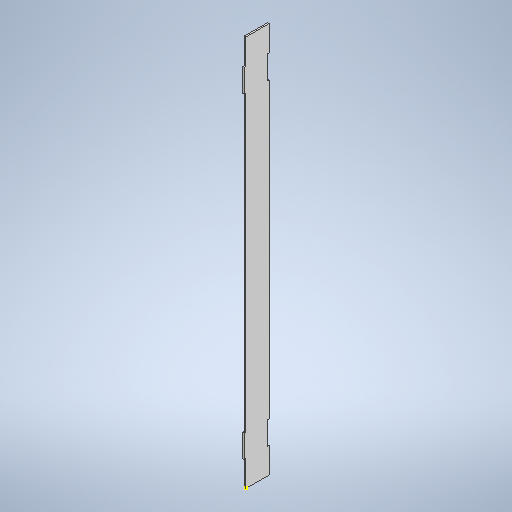
# Autodesk Inventor part: PAREDES LAT-CONTRA
Saved by Autodesk Inventor 2025.2 (Build 292293000, 293)
## iProperties
Created: 2025-05-13
Part Number: PAREDES LAT-CONTRA
Material: Genérico
Document SubType Name: Modeling
Designer: marce
Density: 1 g/cm^3
Appearance: Padrão
Author: marce
Autodesk Inventor part; units mm, degrees
ref_plane "YZ Plane" through (0, 0, 0) normal (1, 0, 0) x (0, 1, 0)
ref_plane "XZ Plane" through (0, 0, 0) normal (0, 1, 0) x (-1, 0, 0)
ref_plane "XY Plane" through (0, 0, 0) normal (0, 0, 1) x (1, 0, 0)
sketch "Esboço1" plane through (0, 0, 0) normal (1, 0, 0) x (0, 1, 0)
  line L0 (1008, 0) -> (1008, -60)
  line L1 (0, -60) -> (0, 0)
  line L2 (1008, 0) -> (942, 0)
  line L3 (942, 0) -> (942, 4)
  line L4 (942, 4) -> (882, 4)
  line L5 (882, 4) -> (882, 0)
  line L6 (0, 0) -> (66, 0)
  line L7 (66, 0) -> (66, 4)
  line L8 (66, 4) -> (126, 4)
  line L9 (126, 4) -> (126, 0)
  line L10 (126, 0) -> (882, 0)
  line L11 (1008, -60) -> (942, -60)
  line L12 (942, -60) -> (942, -56)
  line L13 (942, -56) -> (882, -56)
  line L14 (882, -56) -> (882, -60)
  line L15 (0, -60) -> (66, -60)
  line L16 (66, -60) -> (66, -56)
  line L17 (66, -56) -> (126, -56)
  line L18 (126, -56) -> (126, -60)
  line L19 (126, -60) -> (882, -60)
  dimension "d0" = 1008
  dimension "d1" = 60
  dimension "d4" = 66
  dimension "d5" = 4
  dimension "d6" = 60
  dimension "d7" = 66
  dimension "d8" = 4
  dimension "d9" = 60
  dimension "d10" = 4
  dimension "d11" = 60
  dimension "d12" = 4
  dimension "d13" = 4
  constraints: 40 end point, 11 perpendicular, 4 horizontal, 2 point on line, 2 vertical, 1 parallel
  measures "d0" distance of L0.end L1.start
  measures "d1" distance of L0.start L0.end
  measures "d4" distance of L0.start L2.end
  measures "d5" distance of L2.end L3.end
  measures "d6" distance of L3.end L4.end
  measures "d7" distance of L1.end L6.end
  measures "d8" distance of L6.end L7.end
  measures "d9" distance of L7.end L8.end
  measures "d10" distance of L11.end L12.end
  measures "d11" distance of L12.end L13.end
  measures "d12" distance of L13.end L14.end
  measures "d13" distance of L15.end L16.end
extrude "Extrusão1" add sketch "Esboço1" along normal blind 4
sketch "Esboço2" plane through (4, 0, 0) normal (1, 0, 0) x (0, 0, -1)
  point P0 (0, 0)
